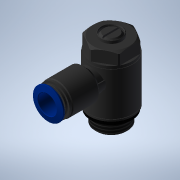
# Autodesk Inventor part: 193152 GRLA-1/2-QS-12-D
Saved by Autodesk Inventor 2021 (Build 250183000, 183)
## iProperties
Created: 2025-06-11
Part Number: 193152 GRLA-1/2-QS-12-D
Material: Generic
Catalog Web Link: www.cadenas.de
Description: GRLA-D-one-way flow control valve
Vendor: FESTO
Document SubType Name: Modeling
Designer: psAdmin
Manufacturer: FESTO
Mass: 106 g
Surface Area: 96.6687 cm^2
Volume: 29.9419 cm^3
Density: 1 g/cm^3
Appearance: PSOLRGB-175-175-175
Category: PARTsolutions
Company: FESTO
Title: 193152 GRLA-1/2-QS-12-D
Author: Cadenas PARTsolutions
Comments: one-way flow control valve
PSOL_IDENT_0: {$CADENAS_DATA/23d-libs/festo/parts/g/grla/grla_d.prj},187 {VTYP=3D},{NB=193152 GRLA-1/2-QS-12-D},{L
PSOL_IDENT_1: INA=193152 GRLA-1/2-QS-12-D},{NN=GRLA-D},{DATE=02.05.2025 09:35:38},{GEOMDATE=20.03.2025 09:32:41},{
PSOL_IDENT_2: VERSION=},{LINEID=140},{WBVAR=},{WBNUMERIC=}  {NB=193152 GRLA-1/2-QS-12-D},{LINA=193152 GRLA-1/2-QS-
PSOL_IDENT_3: 12-D},{KT=DUMMY},{TNR=193152},{TYP=GRLA-1/2-QS-12-D},{INFO=},{FDTQS=12},{FDTQSV2=12},{FDTQS1=-},{FDT
PSOL_IDENT_4: QS2=-},{FDTQSDGST=-},{ZOLL=1/2},{VERS=1.000},{D=G1/2},{QS=QS-12},{ESTE=-},{DFC=-},{B=0.000},{DP=20.9
PSOL_IDENT_5: 55},{KDRD=18.613},{D1=27.800},{D2=20.500},{DS=12.000},{H=55.300},{H1=41.400},{L=42.600},{L1=8.350},{
PSOL_IDENT_6: L2=22.750},{SW=24.000},{CNSMASSEXACT=0.10600},{MOM=15 ±1.5},{GB=2.350},{LHT=1.900},{TW=1.100},{DW=27
PSOL_IDENT_7: .800},{DHT=13.400},{DCH=23.500},{DH=27.200},{HH=9.400},{HHB=11.100},{DI=8.000},{DIH=12.200},{LIH=0.5
PSOL_IDENT_8: 30},{LTS=9.344},{DSJ1=15.000},{DSJ2=16.000},{TSJ=5.000},{LSJ1=15.700},{LSJ2=36.800},{ASJ=45.000},{LS
PSOL_IDENT_9: J3=2.915},{LSJ4=0.000},{LSJ5=4.100},{LSJ6=0.100},{DSJ3=12.200},{DSJ4=19.800},{DQS=0.000},{LQS=0.000}
PSOL_IDENT_10: ,{DSJ5=17.400},{RSJ1=0.200},{RSJ2=0.300},{DSJ6=15.000},{DSR=26.450},{TSR=2.350},{DSJ7=19.800},{HN=0.
PSOL_IDENT_11: 000},{DN=0.000},{DIN=0.000},{DNC=0.000},{CHN=0.000},{RN=0.000},{HKH=0.000},{DKH=0.000},{DIKH=0.000},
PSOL_IDENT_12: {DKHC=0.000},{CHKH=0.000},{CHKH1=0.000},{RKH=0.000},{TKHS=0.000},{HSJ=0.000},{HSJN=0.000},{DAS=0.000
PSOL_IDENT_13: },{TIH=2.000},{SRGH=0.300},{DISR=25.500},{TQS=23.500},{EOLDATE=},{GTIN=4052568015114},{REACH=Ja},{RE
PSOL_IDENT_14: ACHSVHC=Nein},{REACHHAZSUBS=-},{REACHSCIP=-},{REACHVALDATE=-}
NB: 193152 GRLA-1/2-QS-12-D
NN: GRLA-D
NT: one-way flow control valve
NBSYN: $TNR. $TYP.
LINA: 193152 GRLA-1/2-QS-12-D
CATALOG: Festo
TNR: 193152
TYP: GRLA-1/2-QS-12-D
D: G1/2
QS: QS-12
ESTE: -
DFC: -
B: 0
D1: 27.8
D2: 20.5
DS: 12
H: 55.3
H1: 41.4
L: 42.6
L1: 8.35
L2: 22.75
SW: 24
CNSMASSEXACT: 0.106
MOM: 15 ±1.5
GTIN: 4052568015114
REACH: Yes
REACHSVHC: No
REACHHAZSUBS: -
REACHSCIP: -
REACHVALDATE: -
SUPPLIER: FESTO
ARTICLENO: 193152 GRLA-1/2-QS-12-D
BOMINFO: 193152 GRLA-1/2-QS-12-D
CREATOR: CADENAS GmbH
Autodesk Inventor part; units mm, degrees
sketch "Sketch_19" plane through (0, 0, 0) normal (1, 0, 0) x (0, 1, 0)
  line L0 (-31.1, 0) -> (19.85, 0)
  line L1 (19.85, 0) -> (19.85, -4.672)
  line L2 (19.85, -4.672) -> (17.95, -6.1)
  line L3 (17.95, -6.1) -> (19.32, -6.1)
  line L4 (19.32, -6.1) -> (19.85, -6.3471)
  line L5 (19.85, -6.3471) -> (19.85, -6.5)
  line L6 (19.85, -6.5) -> (19.65, -6.7)
  line L7 (19.65, -6.7) -> (17.95, -6.7)
  line L8 (17.95, -6.7) -> (17.95, -11.75)
  line L9 (17.95, -11.75) -> (16.8819, -13.6)
  line L10 (16.8819, -13.6) -> (8.75, -13.6)
  line L11 (8.75, -13.6) -> (8.75, -13.9)
  line L12 (8.75, -13.9) -> (-19, -13.9)
  line L13 (-19, -13.9) -> (-19, -13.05)
  arc A0 (-19, -13.05) -> (-19.3, -13.35) centre (-19, -13.35) ccw
  line L14 (-19.3, -13.35) -> (-19.3, -13.9)
  line L15 (-19.3, -13.9) -> (-20.4, -13.9)
  line L16 (-20.4, -13.9) -> (-20.4, -13.225)
  line L17 (-20.4, -13.225) -> (-22.75, -13.225)
  line L18 (-22.75, -13.225) -> (-22.75, -10.4775)
  line L19 (-22.75, -10.4775) -> (-29.938, -10.4775)
  line L20 (-29.938, -10.4775) -> (-31.1, -9.3155)
  line L21 (-31.1, -9.3155) -> (-31.1, 0)
  line L22 (-31.1, 0) -> (19.85, 0)
  constraints: 46 end point, 2 point on circle, 1 centre point
revolve "Revolution1" add sketch "Sketch_19" angle 360 about axis through (0, -31.1, 0) along (0, -1, 0)
thread "Thread1" size "G20.955x1.814" designation "G 1/2" class "A" standard "ISO Pipe Threads" full length
sketch "Sketch_15" plane through (0, 19.85, 0) normal (0, 1, 0) x (1, 0, 0)
  line L0 (-24, -13.8564) -> (0, -27.7128)
  line L1 (0, -27.7128) -> (24, -13.8564)
  line L2 (24, -13.8564) -> (24, 13.8564)
  line L3 (24, 13.8564) -> (0, 27.7128)
  line L4 (0, 27.7128) -> (-24, 13.8564)
  line L5 (-24, 13.8564) -> (-24, -13.8564)
  line L6 (-12, -6.9282) -> (0, -13.8564)
  line L7 (0, -13.8564) -> (12, -6.9282)
  line L8 (12, -6.9282) -> (12, 6.9282)
  line L9 (12, 6.9282) -> (0, 13.8564)
  line L10 (0, 13.8564) -> (-12, 6.9282)
  line L11 (-12, 6.9282) -> (-12, -6.9282)
  constraints: 24 end point
extrude "Extrusion1" cut sketch "Sketch_15" against normal blind 9.4
sketch "Sketch_16" plane through (0, 19.85, 0) normal (0, 1, 0) x (1, 0, 0)
  line L0 (-0.55, 5.9747) -> (-0.55, -5.9747)
  arc A0 (-0.55, -5.9747) -> (0.55, -5.9747) centre (0, 0) ccw
  line L1 (0.55, -5.9747) -> (0.55, 5.9747)
  arc A1 (0.55, 5.9747) -> (-0.55, 5.9747) centre (0, 0) ccw
  constraints: 4 end point, 4 point on circle, 2 centre point
extrude "Extrusion2" cut sketch "Sketch_16" against normal blind 1.2
sketch "Sketch_17" plane through (0, 0, 0) normal (1, 0, 0) x (0, 1, 0)
  line L0 (0, 0) -> (0, 41.4)
  line L1 (0, 41.4) -> (6.3, 41.4)
  line L2 (6.3, 41.4) -> (9.7347, 40.7944)
  arc A0 (9.9, 40.5974) -> (9.7347, 40.7944) centre (9.7, 40.5974) ccw
  line L3 (9.9, 40.5974) -> (9.9, 39.9)
  line L4 (9.9, 39.9) -> (7.9, 39.9)
  arc A1 (7.9, 39.9) -> (7.5, 39.5) centre (7.9, 39.5) ccw
  line L5 (7.5, 39.5) -> (7.5, 38.085)
  line L6 (7.5, 38.085) -> (8.6, 38.085)
  line L7 (8.6, 38.085) -> (8.7, 37.985)
  line L8 (8.7, 37.985) -> (8.7, 36.8)
  line L9 (8.7, 36.8) -> (9.9, 36.8)
  line L10 (9.9, 36.8) -> (9.9, 35.3)
  line L11 (9.9, 35.3) -> (10.25, 34.6938)
  line L12 (10.25, 34.6938) -> (10.25, 18.45)
  line L13 (10.25, 18.45) -> (7.5, 15.7)
  line L14 (7.5, 15.7) -> (7.5, 0)
  line L15 (7.5, 0) -> (0, 0)
  line L16 (0, 0) -> (0, 41.4)
  constraints: 34 end point, 4 point on circle, 2 centre point
revolve "Revolution2" add sketch "Sketch_17" angle 360 about axis through (0, 0, 0) along (0, 0, -1)
sketch "Sketch_18" plane through (0, 0, 0) normal (0, 0, 1) x (1, 0, 0)
  arc A0 (-7.5993, 2.5) -> (-7.5993, -2.5) centre (0, 0) ccw
  line L0 (-7.5993, -2.5) -> (7.5993, -2.5)
  arc A1 (7.5993, -2.5) -> (7.5993, 2.5) centre (0, 0) ccw
  line L1 (7.5993, 2.5) -> (-7.5993, 2.5)
  constraints: 4 end point, 4 point on circle, 2 centre point
extrude "Extrusion3" add sketch "Sketch_18" along normal blind 20.7
sketch "Sketch_5" plane through (0, 0, 0) normal (1, 0, 0) x (0, 1, 0)
  line L0 (0, 0) -> (0, 41.4)
  line L1 (0, 41.4) -> (6.3, 41.4)
  arc A0 (6.3, 41.4) -> (6, 41.1) centre (6.3, 41.1) ccw
  line L2 (6, 41.1) -> (6, 17.9)
  line L3 (6, 17.9) -> (3, 17.9)
  line L4 (3, 17.9) -> (3, 0)
  line L5 (3, 0) -> (0, 0)
  line L6 (0, 0) -> (0, 41.4)
  constraints: 14 end point, 2 point on circle, 1 centre point
revolve "Revolution3" cut sketch "Sketch_5" angle 360 about axis through (0, 0, 0) along (0, 0, -1)
sketch "Sketch7" plane through (0, -31.1, 0) normal (0, -1, 0) x (1, 0, 0)
  point P0 (0, 0)
hole "Hole1" at (0, -31.1, 0) direction (0, 1, 0) diameter 8 depth 37.1 countersink diameter 8.3464 countersink angle 60
ref_plane "FDT_MOUNT_XY" through (0, -22.75, 0) normal (0, 1, 0) x (-1, 0, 0)
ref_plane "FDT_MOUNT_YZ" through (0, -22.75, 0) normal (-1, 0, 0) x (0, 0, 1)
ref_plane "FDT_MOUNT_ZX" through (0, -22.75, 0) normal (0, 0, 1) x (0, 1, 0)
ref_plane "FDT_SCHLAUCH_XY" through (0, 0, 17.9) normal (0, 0, 1) x (1, 0, 0)
ref_plane "FDT_SCHLAUCH_YZ" through (0, 0, 17.9) normal (1, 0, 0) x (0, 1, 0)
ref_plane "FDT_SCHLAUCH_ZX" through (0, 0, 17.9) normal (0, 1, 0) x (0, 0, 1)
ref_plane "Zylinder_XY" through (0, -31.1, 0) normal (0, 1, 0) x (1, 0, 0)
ref_plane "Zylinder_YZ" through (0, -31.1, 0) normal (1, 0, 0) x (0, 0, -1)
ref_plane "Zylinder_ZX" through (0, -31.1, 0) normal (0, 0, -1) x (0, 1, 0)
ref_plane "anbau_XY" through (0, -22.75, 0) normal (0, 1, 0) x (1, 0, 0)
ref_plane "anbau_YZ" through (0, -22.75, 0) normal (1, 0, 0) x (0, 0, -1)
ref_plane "anbau_ZX" through (0, -22.75, 0) normal (0, 0, -1) x (0, 1, 0)
body "Solid1"
